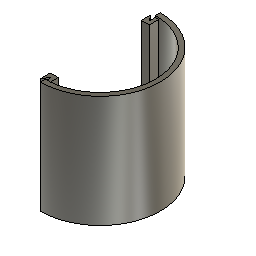
base_side v20 (Autodesk Fusion 360 design; units mm, degrees)
Autodesk Fusion 360 part; units mm, degrees
note: some values were not read from the file. Set by a fixed rule: which sketch regions a step uses.
sketch "Sketch4" plane through (0, 0, 0) normal (0, 0, 1) x (1, 0, 0)
  line L0 (0, 37.5) -> (0, -37.5)
  line L1 (0, 0) -> (37.5, 0)
  arc A0 (0, -34.5) -> (0, 34.5) centre (0, 0) ccw
  arc A1 (0, -37.5) -> (0, 37.5) centre (0, 0) ccw
  line L2 (0, 37.5) -> (-2.5, 37.5) construction
  line L3 (0, 34.5) -> (0, 30.5)
  line L4 (0, 30.5) -> (-2.8008, 34.5)
  line L5 (-2.8008, 34.5) -> (-2.8008, 28.5)
  line L6 (-2.8008, 28.5) -> (2.1992, 28.5)
  line L7 (2.1992, 28.5) -> (2.1992, 34.4298)
  line L8 (2.1992, -28.5) -> (2.1992, -34.4298)
  line L9 (0, -34.5) -> (0, -30.5)
  line L10 (0, -30.5) -> (-2.8008, -34.5)
  line L11 (-2.8008, -34.5) -> (-2.8008, -28.5)
  line L12 (-2.8008, -28.5) -> (2.1992, -28.5)
  dimension "d10" = 75
  dimension "d20" = 4
  dimension "d21" = 35
  dimension "d23" = 5
  dimension "d29" = 2
  dimension "d30" = 6
  dimension "d36" = 3
  constraint coincident L1.start A0.centre
  constraint vertical L0
  constraint coincident L1.end A1
  constraint perpendicular L0 L1
  constraint coincident L0 A0.start
  constraint tangent A1 L2
  constraint parallel L0 L3
  constraint parallel L3 L5
  constraint perpendicular L3 L6
  constraint coincident A0 L7.end
  constraint perpendicular L6 L7
  constraint coincident L0 L3.end
  constraint symmetric L1 A0.end A0.start
  constraint symmetric L1 L3.end L9.end
  constraint symmetric L1 L4.end L10.end
  constraint symmetric L1 L5.end L11.end
  constraint symmetric L1 L6.end L8.start
  constraint symmetric L1 L7.end L8.end
  measures "d10" diameter of A1
  measures "d20" distance of A0.end L3.end
  measures "d21" angle of L3 L4
  measures "d23" distance of L5.end L6.end
  measures "d29" distance of L3.end L6
  measures "d30" distance of L4.end L5.end
  measures "d36" distance of A0 A1
extrude "Extrude6" add sketch "Sketch4" along normal blind 70 contours L0 L1 A0 A1 | L0 A0 L3 L6 L7 | L0 L1 A0 A1 | L0 L4 L5 L6 | L0 A0 L8 L9 L12 | L0 L10 L11 L12 makes body 1
sketch "Sketch6" plane through (0, 0, 70) normal (0, 0, 1) x (-1, 0, 0)
  arc A0 (0, 37.5) -> (0, -37.5) centre (0, 0) ccw
  line L0 (0, 30.5) -> (0, 37.5)
  line L1 (0, -30.5) -> (2.8008, -34.5)
  line L2 (2.8008, -34.5) -> (2.8008, -28.5)
  line L3 (2.8008, -28.5) -> (-2.1992, -28.5)
  line L4 (0, 37.5) -> (0, -28.5)
  line L5 (0, -28.5) -> (2.8008, -28.5)
  line L6 (0, -30.5) -> (0, -28.5)
  line L7 (2.8008, -28.5) -> (2.8008, -34.5)
  line L8 (-2.1992, -31.9243) -> (-2.1992, -26)
  line L9 (-2.1992, -31.9243) -> (0, -31.9243)
  line L10 (-2.1992, -28.5) -> (-2.1992, -34.4298)
  arc A1 (-2.1992, 34.4298) -> (-2.1992, -34.4298) centre (0, 0) ccw
  line L11 (-2.1992, 34.4298) -> (-2.1992, 28.5)
  line L12 (-2.1992, 28.5) -> (2.8008, 28.5)
  line L13 (2.8008, 28.5) -> (2.8008, 34.5)
  line L14 (2.8008, 34.5) -> (0, 30.5)
  line L15 (0, -37.5) -> (0, -30.5)
  arc A2 (2.7253, -34.3922) -> (2.8008, -34.3861) centre (0, 0) ccw
  arc A3 (2.8008, 34.3861) -> (2.7253, 34.3922) centre (0, 0) ccw
  arc A4 (0, 34.5) -> (-2.1992, 34.4298) centre (0, 0) ccw
  arc A5 (-2.1992, -34.4298) -> (0, -34.5) centre (0, 0) ccw
  constraint coincident A0.start L0.end
  constraint coincident L3 L4.end
  constraint perpendicular L3 L4
  constraint coincident L2.end L3.start
  constraint coincident L1.start L6.start
  constraint coincident L1.end L2.start
  constraint coincident A0.centre A1.centre
  constraint coincident L10.end A3
  constraint coincident L2 A2.end
  constraint coincident L13 A3.start
  constraint coincident L15 A5.end
  constraint coincident L1 A2.start
  constraint concentric A2 A3
  constraint coincident L14 A3.end
  constraint coincident L0 A4.start
  constraint concentric A3 A4
  constraint concentric A4 A5
extrude "Extrude7" cut sketch "Sketch6" against normal blind 1 contours L0 L4 L11 L12 A4 | L9 L10 L15 A5 | L4 L12 L13 L14 A3 | L3 L6 L8 L9 L10 L15 | L13 L14 A3 | L1 L2 L3 L5 L6 L7 A2 | L1 L2 L7 A2 bodies 1
mirror "Mirror2" about plane through (0, 0, 0) normal (0, 1, 0) of "Extrude7"
sketch "Sketch7" plane through (0, 0, 69) normal (0, 0, 1) x (-1, 0, 0)
  line L0 (2.8008, -34.5) -> (2.8008, -28.5)
  line L1 (2.8008, -28.5) -> (-2.1992, -28.5)
  line L2 (2.8008, -34.5) -> (2.8008, -28.5)
  line L3 (0, -30.5) -> (2.8008, -34.5)
  line L4 (0, -30.5) -> (2.8008, -34.5)
  line L5 (2.7008, -28.5) -> (2.7008, -34.1828)
  line L6 (2.7008, -34.1828) -> (0, -30.3257)
  line L7 (0, -30.5) -> (0, -30.3257)
  arc A0 (-2.1992, -34.4298) -> (0, -34.5) centre (0, 0) ccw
  dimension "d37" = 0.1
  dimension "d38" = 0.1
  constraint coincident L1 L5.start
  constraint perpendicular L1 L5
  constraint parallel L4 L6
  constraint coincident L3.start L4.start
  constraint vertical L7
  measures "d37" distance of L2 L5.end
  measures "d38" distance of L3 L6
extrude "Extrude8" cut sketch "Sketch7" against normal blind 70 bodies 1
mirror "Mirror3" about plane through (0, 0, 0) normal (0, 1, 0) of "Extrude6", "Extrude7", "Mirror2", "Extrude8" makes body 2
fillet "Fillet1" radius 0.2 4 edges at (-2.7008, 34.1828, 34.5) (0, 30.3257, 34.5) (-2.7008, -34.1828, 34.5) (0, -30.3257, 34.5) on bodies 1 2
combine "Combine1" operation add target body 2 tool bodies 1
